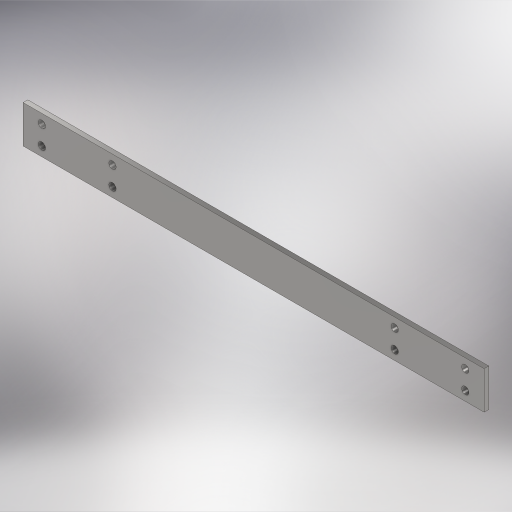
# Autodesk Inventor part: Chassis Bar
Saved by Autodesk Inventor 2024 (Build 280153000, 153)
## iProperties
Created: 2023-11-09
Part Number: Chassis Bar
Material: Stainless Steel
Document SubType Name: Modeling
Designer: aaron
Density: 8 g/cm^3
Appearance: Semi-Polished
Author: aaron
Autodesk Inventor part; units mm, degrees
ref_plane "YZ Plane" through (0, 0, 0) normal (1, 0, 0) x (0, 1, 0)
ref_plane "XZ Plane" through (0, 0, 0) normal (0, 1, 0) x (-1, 0, 0)
ref_plane "XY Plane" through (0, 0, 0) normal (0, 0, 1) x (1, 0, 0)
sketch "Sketch1" plane through (0, 0, 0) normal (0, 0, 1) x (1, 0, 0)
  line L0 (155.575, 12.7) -> (-155.575, 12.7)
  line L1 (-155.575, 12.7) -> (-155.575, -12.7)
  line L2 (-155.575, -12.7) -> (155.575, -12.7)
  line L3 (155.575, -12.7) -> (155.575, 12.7)
  line L4 (155.575, 12.7) -> (-155.575, -12.7) construction
  line L5 (-155.575, 12.7) -> (155.575, -12.7) construction
  line L6 (-149.225, 12.7) -> (-136.525, 12.7)
  line L7 (-136.525, 12.7) -> (-136.525, -12.7)
  line L8 (-136.525, -12.7) -> (-149.225, -12.7)
  line L9 (-149.225, -12.7) -> (-149.225, 12.7)
  circle A0 centre (-142.875, 6.35) radius 2.4257
  circle A1 centre (-142.875, -6.35) radius 2.4257
  line L10 (149.225, 12.7) -> (136.525, 12.7)
  line L11 (136.525, 12.7) -> (136.525, -12.7)
  line L12 (136.525, -12.7) -> (149.225, -12.7)
  line L13 (149.225, -12.7) -> (149.225, 12.7)
  circle A2 centre (142.875, 6.35) radius 2.4257
  circle A3 centre (142.875, -6.35) radius 2.4257
  line L14 (101.6, 12.7) -> (88.9, 12.7)
  line L15 (88.9, 12.7) -> (88.9, -12.7)
  line L16 (88.9, -12.7) -> (101.6, -12.7)
  line L17 (101.6, -12.7) -> (101.6, 12.7)
  line L18 (-101.6, 12.7) -> (-88.9, 12.7)
  line L19 (-88.9, 12.7) -> (-88.9, -12.7)
  line L20 (-88.9, -12.7) -> (-101.6, -12.7)
  line L21 (-101.6, -12.7) -> (-101.6, 12.7)
  circle A4 centre (-95.25, 6.35) radius 2.4257
  circle A5 centre (-95.25, -6.35) radius 2.4257
  circle A6 centre (95.25, -6.35) radius 2.4257
  circle A7 centre (95.25, 6.35) radius 2.4257
  point P0 (0, 0)
  point P1 (149.225, 0)
  dimension "d0" = 311.15
  dimension "d1" = 25.4
  dimension "d2" = 12.7
  dimension "d3" = 6.35
  dimension "d4" = 4.8514
  dimension "d5" = 4.8514
  dimension "d6" = 6.35
  dimension "d7" = 6.35
  dimension "d8" = 12.7
  dimension "d9" = 6.35
  dimension "d10" = 4.8514
  dimension "d11" = 4.8514
  dimension "d12" = 12.7
  dimension "d13" = 47.625
  dimension "d14" = 12.7
  dimension "d15" = 47.625
  dimension "d16" = 4.8514
  dimension "d17" = 4.8514
  dimension "d18" = 4.8514
  dimension "d19" = 4.8514
  dimension "d22" = 6.35
  dimension "d23" = 6.35
  dimension "d24" = 6.35
  dimension "d25" = 6.35
  dimension "d26" = 6.35
  dimension "d27" = 6.35
  dimension "d28" = 6.35
  dimension "d29" = 6.35
  constraints: 44 end point, 10 parallel, 8 centre point, 8 point on line, 5 horizontal, 5 perpendicular, 3 midpoint
  measures "d0" distance of L2.end L1.end
  measures "d1" distance between parallel lines of L0 L2
  measures "d2" distance of L7.end L8.end
  measures "d3" distance between parallel lines of L1 L9
  measures "d4" diameter of A0
  measures "d5" diameter of A1
  measures "d6" distance from line of L2 A1.centre
  measures "d7" distance from line of L0 A0.centre
  measures "d8" distance of L12.end L11.end
  measures "d9" distance between parallel lines of L3 L13
  measures "d10" diameter of A2
  measures "d11" diameter of A3
  measures "d12" distance of L16.end L15.end
  measures "d13" distance between parallel lines of L17 L13
  measures "d14" distance of L19.end L20.end
  measures "d15" distance between parallel lines of L9 L21
  measures "d16" diameter of A4
  measures "d17" diameter of A5
  measures "d18" diameter of A6
  measures "d19" diameter of A7
  measures "d22" distance from line of L9 A1.centre
  measures "d23" distance from line of L9 A0.centre
  measures "d24" distance from line of L21 A5.centre
  measures "d25" distance from line of L21 A4.centre
  measures "d26" distance from line of L13 A3.centre
  measures "d27" horizontal distance of point (149.225, 0) A2.centre
  measures "d28" distance from line of L17 A6.centre
  measures "d29" distance from line of L17 A7.centre
extrude "Extrusion1" add sketch "Sketch1" along normal blind 3.175
body "Solid1"
